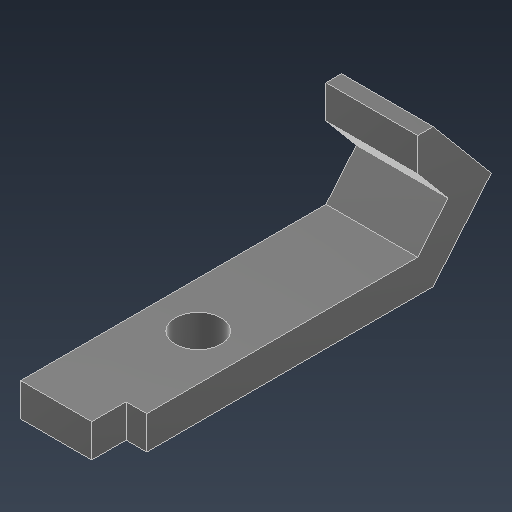
# Autodesk Inventor part: Cap Pulley Support V2 Pt1
Saved by Autodesk Inventor 2021.3 (Build 253353000, 353)
## iProperties
Created: 2022-07-27
Part Number: Cap Pulley Support V2 Pt1
Material: Thermoplastic Resin
Document SubType Name: Modeling
Designer: david
Density: 1.28 g/cm^3
Appearance: Smooth - Black
Author: david
Autodesk Inventor part; units mm, degrees
ref_plane "YZ Plane" through (0, 0, 0) normal (1, 0, 0) x (0, 1, 0)
ref_plane "XZ Plane" through (0, 0, 0) normal (0, 1, 0) x (-1, 0, 0)
ref_plane "XY Plane" through (0, 0, 0) normal (0, 0, 1) x (1, 0, 0)
sketch "Sketch1" plane through (0, 0, 0) normal (1, 0, 0) x (0, 1, 0)
  line L0 (0, 0) -> (2.9, 0)
  line L1 (2.9, 0) -> (2.9, -25)
  line L2 (2.9, -25) -> (0, -25)
  line L3 (0, -25) -> (0, 0)
  line L4 (0, -25) -> (6.05, -30.0766)
  line L5 (2.9, -23.6477) -> (6.05, -26.2909)
  line L6 (6.05, -30.0766) -> (6.05, -26.2909)
  line L7 (6.05, -26.2909) -> (9.2, -23.6477)
  line L8 (6.05, -30.0766) -> (12.1, -25)
  line L9 (9.2, -27.4334) -> (9.2, -23.6477)
  line L10 (7.5884, -25) -> (12.1, -25)
  line L11 (12.1, -25) -> (12.1, -23.6477)
  line L12 (12.1, -23.6477) -> (9.2, -23.6477)
  dimension "d0" = 2.9
  dimension "d1" = 25
  dimension "d2" = 50
  dimension "d3" = 3.15
  dimension "d4" = 2.9
  dimension "d5" = 50
  dimension "d6" = 3.15
  constraints: 26 end point, 5 point on line, 4 parallel, 3 perpendicular, 2 vertical, 1 horizontal
  measures "d0" distance of L0.start L0.end
  measures "d1" distance between parallel lines of L0 L2
  measures "d2" angle of L3 L4
  measures "d3" distance from line of L1 L4.end
  measures "d4" distance between parallel lines of L4 L5
  measures "d5" angle of L6 L7
  measures "d6" distance between parallel lines of L6 L9
extrude "Extrusion1" add sketch "Sketch1" along normal blind 8
sketch "Sketch2" plane through (0, 0, 0) normal (0, 0, 1) x (1, 0, 0)
  line L0 (0, 0) -> (8, 0) projected
  line L1 (0, 0) -> (6.2, 0)
  line L2 (6.2, 0) -> (6.2, 2.9)
  line L3 (6.2, 2.9) -> (0, 2.9)
  line L4 (0, 2.9) -> (0, 0)
  dimension "d11" = 6.2
  constraints: 8 end point, 2 parallel, 1 perpendicular, 1 point on line
  measures "d11" distance of L2.end L3.end
extrude "Extrusion2" add sketch "Sketch2" along normal blind 3
sketch "Sketch3" plane through (0, 2.9, -23.6477) normal (0, 1, 0) x (1, 0, 0)
  line L0 (6.2, -23.6477) -> (8, -23.6477) projected
  line L1 (0, -23.6477) -> (8, -23.6477)
  line L2 (4, -23.6477) -> (4, -15.1477)
  circle A0 centre (4, -15.1477) radius 2
  dimension "d14" = 8.5
  dimension "d15" = 4
  constraints: 4 end point, 1 centre point, 1 coincident, 1 horizontal, 1 midpoint, 1 vertical
  measures "d14" distance of L2.start L2.end
  measures "d15" diameter of A0
extrude "Extrusion3" cut sketch "Sketch3" against normal through all
equation "\"d6\" = d3"
body "Solid1"
